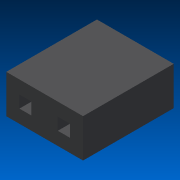
# Autodesk Inventor part: jumper
Saved by Autodesk Inventor 2015 SP1 (Build 190203100, 203)
## iProperties
Created: 2015-12-01
Part Number: jumper
Material: Generic
Document SubType Name: Modeling
Designer: User
Density: 1 g/cm^3
Appearance: Default
Author: User
Autodesk Inventor part; units mm, degrees
ref_plane "YZ Plane" through (0, 0, 0) normal (1, 0, 0) x (0, 1, 0)
ref_plane "XZ Plane" through (0, 0, 0) normal (0, 1, 0) x (-1, 0, 0)
ref_plane "XY Plane" through (0, 0, 0) normal (0, 0, 1) x (1, 0, 0)
sketch "Эскиз1" plane through (0, 0, 0) normal (0, 1, 0) x (-1, 0, 0)
  line L0 (2.54, -1.27) -> (-2.54, -1.27)
  line L1 (-2.54, -1.27) -> (-2.54, 1.27)
  line L2 (-2.54, 1.27) -> (2.54, 1.27)
  line L3 (2.54, 1.27) -> (2.54, -1.27)
  line L4 (0, -1.778) -> (0, 1.778) projected
  line L5 (3.556, 0) -> (-3.556, 0) projected
  point P0 (0, 0)
  dimension "d0" = 5.08
  dimension "d1" = 2.54
  constraints: 8 end point, 2 parallel, 1 horizontal, 1 perpendicular, 2 other
  measures "d0" distance of L1.end L2.end
  measures "d1" distance of L0.end L1.end
extrude "Выдавливание1" add sketch "Эскиз1" along normal blind 6
sketch "Эскиз2" plane through (0, 6, 0) normal (0, 1, 0) x (1, 0, 0)
  line L0 (-1.67, 0.4) -> (-0.87, 0.4)
  line L1 (-0.87, 0.4) -> (-0.87, -0.4)
  line L2 (-0.87, -0.4) -> (-1.67, -0.4)
  line L3 (-1.67, -0.4) -> (-1.67, 0.4)
  line L4 (-3.556, 0) -> (3.556, 0) projected
  line L5 (0, 1.778) -> (0, -1.778) projected
  line L6 (0.87, 0.4) -> (1.67, 0.4)
  line L7 (1.67, 0.4) -> (1.67, -0.4)
  line L8 (1.67, -0.4) -> (0.87, -0.4)
  line L9 (0.87, -0.4) -> (0.87, 0.4)
  point P0 (0, 0)
  dimension "d4" = 0.8
  dimension "d5" = 0.8
  dimension "d8" = 2.54
  constraints: 16 end point, 2 horizontal, 2 parallel, 1 collinear, 1 perpendicular, 9 other
  measures "d4" distance of L0.start L0.end
  measures "d5" distance of L2.end L0.start
  measures "d8" distance of L0.start L6.start
extrude "Выдавливание2" cut sketch "Эскиз2" against normal blind 6
